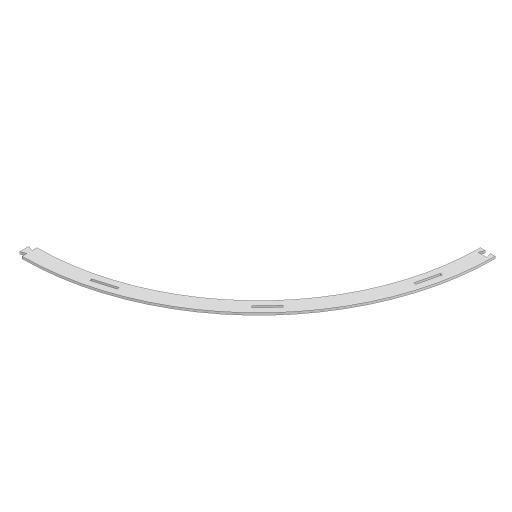
# Autodesk Inventor part: R60_CM_CIRCULO
Saved by Autodesk Inventor 2024.2 (Build 282272000, 272)
## iProperties
Created: 2024-10-01
Part Number: R60_CM_CIRCULO
Material: Generic
Document SubType Name: Modeling
Designer: jrcer
Density: 1 g/cm^3
Appearance: Default
Author: jrcer
Autodesk Inventor part; units mm, degrees
ref_plane "YZ Plane" through (0, 0, 0) normal (1, 0, 0) x (0, 1, 0)
ref_plane "XZ Plane" through (0, 0, 0) normal (0, 1, 0) x (-1, 0, 0)
ref_plane "XY Plane" through (0, 0, 0) normal (0, 0, 1) x (1, 0, 0)
sketch "Sketch1" plane through (0, 0, 0) normal (0, 1, 0) x (-1, 0, 0)
  circle A0 centre (0, 0) radius 300
  circle A1 centre (0, 0) radius 320
  line L0 (320, 0) -> (300, 0)
  line L1 (-320, 0) -> (-300, 0)
  line L2 (0, 0) -> (-300, 0) construction
  line L3 (0, 300) -> (0, 0) construction
  line L4 (0, 320) -> (0, 300)
  line L5 (-300, 0) -> (-320, 0)
  line L6 (-304, 7) -> (-316, 7)
  line L7 (-316, 7) -> (-313.4522, 0)
  line L8 (-304, 7) -> (-306.5478, 0)
  line L9 (-310, 0) -> (-310, 7) construction
  line L10 (-306.201, 57.7437) -> (-299.2289, 86.9223)
  line L11 (-299.2289, 86.9223) -> (-296.1165, 86.1786)
  line L12 (-296.1165, 86.1786) -> (-303.0886, 57)
  line L13 (-303.0886, 57) -> (-306.201, 57.7437)
  line L14 (-306.201, 57.7437) -> (-296.1165, 86.1786) construction
  line L15 (-299.2289, 86.9223) -> (-303.0886, 57) construction
  circle A2 centre (0, 0) radius 310 construction
  line L16 (-7, -304) -> (0, -306.5478)
  line L17 (-7, -316) -> (0, -313.4522)
  line L18 (-7, -304) -> (-7, -316)
  line L19 (304, -7) -> (306.5478, 0)
  line L20 (316, -7) -> (313.4522, 0)
  line L21 (304, -7) -> (316, -7)
  line L22 (7, 304) -> (0, 306.5478)
  line L23 (7, 316) -> (0, 313.4522)
  line L24 (7, 304) -> (7, 316)
  line L25 (-294.0497, -103.093) -> (-302.6009, -74.3375)
  line L26 (-290.9825, -102.1809) -> (-294.0497, -103.093)
  line L27 (-299.5337, -73.4254) -> (-290.9825, -102.1809)
  line L28 (-302.6009, -74.3375) -> (-299.5337, -73.4254)
  line L29 (-203.108, -236.306) -> (-224.8913, -215.6787)
  line L30 (-200.9078, -233.9825) -> (-203.108, -236.306)
  line L31 (-222.6911, -213.3551) -> (-200.9078, -233.9825)
  line L32 (-224.8913, -215.6787) -> (-222.6911, -213.3551)
  line L33 (-57.7437, -306.201) -> (-86.9223, -299.2289)
  line L34 (-57, -303.0886) -> (-57.7437, -306.201)
  line L35 (-86.1786, -296.1165) -> (-57, -303.0886)
  line L36 (-86.9223, -299.2289) -> (-86.1786, -296.1165)
  line L37 (103.093, -294.0497) -> (74.3375, -302.6009)
  line L38 (102.1809, -290.9825) -> (103.093, -294.0497)
  line L39 (73.4254, -299.5337) -> (102.1809, -290.9825)
  line L40 (74.3375, -302.6009) -> (73.4254, -299.5337)
  line L41 (236.306, -203.108) -> (215.6787, -224.8913)
  line L42 (233.9825, -200.9078) -> (236.306, -203.108)
  line L43 (213.3551, -222.6911) -> (233.9825, -200.9078)
  line L44 (215.6787, -224.8913) -> (213.3551, -222.6911)
  line L45 (306.201, -57.7437) -> (299.2289, -86.9223)
  line L46 (303.0886, -57) -> (306.201, -57.7437)
  line L47 (296.1165, -86.1786) -> (303.0886, -57)
  line L48 (299.2289, -86.9223) -> (296.1165, -86.1786)
  line L49 (294.0497, 103.093) -> (302.6009, 74.3375)
  line L50 (290.9825, 102.1809) -> (294.0497, 103.093)
  line L51 (299.5337, 73.4254) -> (290.9825, 102.1809)
  line L52 (302.6009, 74.3375) -> (299.5337, 73.4254)
  line L53 (203.108, 236.306) -> (224.8913, 215.6787)
  line L54 (200.9078, 233.9825) -> (203.108, 236.306)
  line L55 (222.6911, 213.3551) -> (200.9078, 233.9825)
  line L56 (224.8913, 215.6787) -> (222.6911, 213.3551)
  line L57 (57.7437, 306.201) -> (86.9223, 299.2289)
  line L58 (57, 303.0886) -> (57.7437, 306.201)
  line L59 (86.1786, 296.1165) -> (57, 303.0886)
  line L60 (86.9223, 299.2289) -> (86.1786, 296.1165)
  line L61 (-103.093, 294.0497) -> (-74.3375, 302.6009)
  line L62 (-102.1809, 290.9825) -> (-103.093, 294.0497)
  line L63 (-73.4254, 299.5337) -> (-102.1809, 290.9825)
  line L64 (-74.3375, 302.6009) -> (-73.4254, 299.5337)
  line L65 (-236.306, 203.108) -> (-215.6787, 224.8913)
  line L66 (-233.9825, 200.9078) -> (-236.306, 203.108)
  line L67 (-213.3551, 222.6911) -> (-233.9825, 200.9078)
  line L68 (-215.6787, 224.8913) -> (-213.3551, 222.6911)
  point P0 (310, 0)
  point P1 (-310, 0)
  point P2 (-301.1588, 71.9611)
  point P3 (-59.267, 304.2818)
  point P4 (-304.6448, 57.3718)
  point P5 (-297.6727, 86.5504)
  point P6 (-7, -310)
  point P7 (310, -7)
  point P8 (7, 310)
  point P9 (-292.5161, -102.6369)
  point P10 (-301.0673, -73.8815)
  point P11 (-202.0079, -235.1442)
  point P12 (-223.7912, -214.5169)
  point P13 (-57.3718, -304.6448)
  point P14 (-86.5504, -297.6727)
  point P15 (102.6369, -292.5161)
  point P16 (73.8815, -301.0673)
  point P17 (235.1442, -202.0079)
  point P18 (214.5169, -223.7912)
  point P19 (304.6448, -57.3718)
  point P20 (297.6727, -86.5504)
  point P21 (292.5161, 102.6369)
  point P22 (301.0673, 73.8815)
  point P23 (202.0079, 235.1442)
  point P24 (223.7912, 214.5169)
  point P25 (57.3718, 304.6448)
  point P26 (86.5504, 297.6727)
  point P27 (-102.6369, 292.5161)
  point P28 (-73.8815, 301.0673)
  point P29 (-235.1442, 202.0079)
  point P30 (-214.5169, 223.7912)
  point P31 (-306.5478, 0)
  point P32 (0, 306.5478)
  point P33 (0, 313.4522)
  point P34 (-313.4522, 0)
  dimension "d0" = 600
  dimension "d1" = 640
  dimension "d4" = 90
  dimension "d5" = 7
  dimension "d6" = 70
  dimension "d8" = 12
  dimension "d13" = 3.2
  dimension "d14" = 30
  dimension "d15" = 50
  dimension "d20" = 620
  dimension "d23" = 360
  dimension "d27" = 360
  constraints: 138 end point, 11 point on circle, 8 midpoint, 3 centre point, 3 coincident, 3 parallel, 2 horizontal, 2 horizontal alignment, 2 perpendicular, 2 point on line, 2 vertical, 1 collinear, 1 equal length, 154 other
  measures "d0" diameter of A0
  measures "d1" diameter of A1
  measures "d4" angle of L2 L3
  measures "d5" distance between parallel lines of L6 L5
  measures "d6" angle of L7 L6
  measures "d8" distance of L6.start L6.end
  measures "d13" distance of L10.end L11.end
  measures "d14" distance of L11.end L12.end
  measures "d15" vertical distance of L12.end L6.start
  measures "d20" diameter of A2
extrude "Extrusion1" add sketch "Sketch1" along normal blind 3 contours A0 L1 L8 L6 L7 A1 L4 | L4 L23 L24 L22
body "Solid1"
